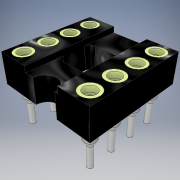
# Autodesk Inventor part: DIL8-Socket
Saved by Autodesk Inventor 2018 (Build 220112000, 112)
## iProperties
Created: 2020-04-18
Part Number: DIL8-Socket
Material: Všeobecné
Document SubType Name: Modeling
Designer: Jozko Mrkvicka
Density: 1 g/cm^3
Appearance: Výchozí
Author: Jozko Mrkvicka
Autodesk Inventor part; units mm, degrees
ref_plane "YZ Plane" through (0, 0, 0) normal (1, 0, 0) x (0, 1, 0)
ref_plane "XZ Plane" through (0, 0, 0) normal (0, 1, 0) x (-1, 0, 0)
ref_plane "XY Plane" through (0, 0, 0) normal (0, 0, 1) x (1, 0, 0)
sketch "Náčrt1" plane through (0, 0, 0) normal (0, 1, 0) x (-1, 0, 0)
  line L0 (10.16, 0) -> (10.16, -10.16)
  line L1 (10.16, -10.16) -> (0, -10.16)
  line L2 (0, -10.16) -> (0, 0)
  line L3 (0, 0) -> (3.175, 0)
  line L4 (3.175, -10.16) -> (0, -10.16)
  line L5 (0, -10.16) -> (0, 0)
  line L6 (10.16, 0) -> (6.985, 0)
  line L7 (6.985, -10.16) -> (10.16, -10.16)
  line L8 (10.16, -10.16) -> (10.16, 0)
  line L9 (3.81, -3.175) -> (6.35, -3.175)
  line L10 (6.985, -10.16) -> (3.175, -10.16)
  line L11 (3.81, -6.985) -> (6.35, -6.985)
  line L12 (6.985, -3.81) -> (6.985, -6.35)
  line L13 (3.175, -3.81) -> (3.175, -6.35)
  arc A0 (3.4925, 0) -> (6.0325, 0) centre (4.7625, 0) ccw
  line L14 (0, 0) -> (3.4925, 0)
  line L15 (6.0325, 0) -> (10.16, 0)
  line L16 (6.985, 0) -> (6.0325, 0)
  line L17 (3.4925, 0) -> (3.175, 0)
  arc A1 (6.985, -3.81) -> (6.35, -3.175) centre (6.35, -3.81) ccw
  arc A2 (3.81, -3.175) -> (3.175, -3.81) centre (3.81, -3.81) ccw
  arc A3 (3.175, -6.35) -> (3.81, -6.985) centre (3.81, -6.35) ccw
  arc A4 (6.35, -6.985) -> (6.985, -6.35) centre (6.35, -6.35) ccw
  dimension "d0" = 10.16
  dimension "d1" = 10.16
  dimension "d6" = 2.54
  dimension "d7" = 0.635
  dimension "d111" = 3.175
  dimension "d112" = 3.175
  constraints: 36 end point, 10 point on circle, 9 parallel, 8 horizontal, 8 tangent, 5 centre point, 4 perpendicular, 3 equal radius, 2 point on line
  measures "d0" distance of L0.end L1.end
  measures "d1" distance of L0.start L0.end
  measures "d6" diameter of A0
  measures "d7" radius of A1
  measures "d111" distance between parallel lines of L1 L11
  measures "d112" distance between parallel lines of L3 L9
extrude "Vysunutí15" add sketch "Náčrt1" along normal blind 3.175
sketch "Náčrt14" plane through (0, 3.175, 0) normal (0, 1, 0) x (1, 0, 0)
  line L0 (-6.985, 11.6552) -> (-3.175, 11.6552)
  line L1 (-3.175, 11.6552) -> (-3.175, -1.5875)
  line L2 (-3.175, -1.5875) -> (-6.985, -1.5875)
  line L3 (-6.985, -1.5875) -> (-6.985, 11.6552)
  point P0 (0, 0)
  constraints: 8 end point, 2 parallel, 1 horizontal, 1 perpendicular
extrude "Vysunutí16" cut sketch "Náčrt14" against normal blind 0.635
sketch "Náčrt15" plane through (0, 3.175, 0) normal (0, 1, 0) x (1, 0, 0)
  circle A0 centre (-8.89, 8.89) radius 0.635
  circle A1 centre (-8.89, 6.35) radius 0.635
  circle A2 centre (-8.89, 3.81) radius 0.635
  circle A3 centre (-8.89, 1.27) radius 0.635
  circle A4 centre (-1.27, 8.89) radius 0.635
  circle A5 centre (-1.27, 6.35) radius 0.635
  circle A6 centre (-1.27, 3.81) radius 0.635
  circle A7 centre (-1.27, 1.27) radius 0.635
  point P0 (0, 0)
  point P1 (0, 0)
  point P2 (-1.27, 8.89)
  point P3 (-1.27, 6.35)
  point P4 (-1.27, 3.81)
  point P5 (-1.27, 1.27)
  point P6 (-8.89, 1.27)
  point P7 (-8.89, 3.81)
  point P8 (-8.89, 6.35)
  point P9 (-8.89, 8.89)
  point P10 (-1.27, 1.27)
  constraints: 8 centre point
extrude "Vysunutí17" cut sketch "Náčrt15" against normal blind 0.635
sketch "Náčrt16" plane through (-8.89, 2.54, -1.27) normal (0, 1, 0) x (1, 0, 0)
  circle A0 centre (0, 7.62) radius 0.3175
  circle A1 centre (0, 7.62) radius 0.3175
  circle A2 centre (7.62, 5.08) radius 0.3175
  circle A3 centre (7.62, 5.08) radius 0.3175
  circle A4 centre (7.62, 2.54) radius 0.3175
  circle A5 centre (7.62, 0) radius 0.3175
  circle A6 centre (7.62, 0) radius 0.3175
  circle A7 centre (0, 5.08) radius 0.3175
  circle A8 centre (0, 2.54) radius 0.3175
  circle A9 centre (0, 0) radius 0.3175
  circle A10 centre (0, 0) radius 0.3175
  circle A11 centre (7.62, 7.62) radius 0.3175
  point P0 (8.89, -1.27)
  point P1 (8.89, -1.27)
  constraints: 12 centre point, 8 coincident
extrude "Vysunutí18" cut sketch "Náčrt16" against normal blind 1.27
sketch "Náčrt17" plane through (0, 3.175, 0) normal (0, 1, 0) x (1, 0, 0)
  circle A0 centre (-8.89, 1.27) radius 0.9525
  circle A1 centre (-8.89, 8.89) radius 0.9525
  circle A2 centre (-8.89, 3.81) radius 0.9525
  circle A3 centre (-8.89, 6.35) radius 0.9525
  circle A4 centre (-1.27, 8.89) radius 0.9525
  circle A5 centre (-1.27, 3.81) radius 0.9525
  circle A6 centre (-1.27, 1.27) radius 0.9525
  circle A7 centre (-1.27, 6.35) radius 0.9525
  point P0 (0, 0)
  constraints: 8 centre point
extrude "Vysunutí19" cut sketch "Náčrt17" against normal blind 0.0254
sketch "Náčrt18" plane through (0, 0, 0) normal (0, -1, 0) x (1, 0, 0)
  circle A0 centre (-1.27, -8.89) radius 0.635 projected
  circle A1 centre (-1.27, -6.35) radius 0.635 projected
  circle A2 centre (-1.27, -3.81) radius 0.635 projected
  circle A3 centre (-1.27, -1.27) radius 0.635 projected
  circle A4 centre (-8.89, -8.89) radius 0.635 projected
  circle A5 centre (-8.89, -6.35) radius 0.635 projected
  circle A6 centre (-8.89, -3.81) radius 0.635 projected
  circle A7 centre (-8.89, -1.27) radius 0.635 projected
  point P0 (0, 0)
extrude "Vysunutí20" add sketch "Náčrt18" along normal blind 1.905
chamfer "Zkosení45" distance 0.3175 distance2 0.635 1 edges at (-9.525, -1.905, -8.89) measured on face at (-8.6783, -1.905, -9.0867)
chamfer "Zkosení46" distance 0.3175 distance2 0.635 1 edges at (-9.525, -1.905, -6.35) measured on face at (-8.6964, -1.905, -6.499)
chamfer "Zkosení47" distance 0.3175 distance2 0.635 1 edges at (-9.525, -1.905, -3.81) measured on face at (-8.6964, -1.905, -3.959)
chamfer "Zkosení48" distance 0.3175 distance2 0.635 1 edges at (-9.525, -1.905, -1.27) measured on face at (-8.6964, -1.905, -1.419)
chamfer "Zkosení49" distance 0.3175 distance2 0.635 1 edges at (-1.905, -1.905, -8.89) measured on face at (-1.4636, -1.905, -8.9377)
chamfer "Zkosení50" distance 0.3175 distance2 0.635 1 edges at (-1.905, -1.905, -6.35) measured on face at (-1.0645, -1.905, -6.4007)
chamfer "Zkosení51" distance 0.3175 distance2 0.635 1 edges at (-1.905, -1.905, -3.81) measured on face at (-1.0282, -1.905, -4.0079)
chamfer "Zkosení52" distance 0.3175 distance2 0.635 1 edges at (-1.905, -1.905, -1.27) measured on face at (-1.0935, -1.905, -1.2787)
sketch "Náčrt19" plane through (-8.89, -1.905, -8.89) normal (0, -1, 0) x (1, 0, 0)
  circle A0 centre (0, 7.62) radius 0.3175 projected
  circle A1 centre (0, 5.08) radius 0.3175 projected
  circle A2 centre (0, 2.54) radius 0.3175 projected
  circle A3 centre (0, 0) radius 0.3175 projected
  circle A4 centre (7.62, 7.62) radius 0.3175 projected
  circle A5 centre (7.62, 5.08) radius 0.3175 projected
  circle A6 centre (7.62, 2.54) radius 0.3175 projected
  circle A7 centre (7.62, 0) radius 0.3175 projected
  point P0 (8.89, 8.89)
extrude "Vysunutí21" add sketch "Náčrt19" along normal blind 2.54
fillet "Zaoblení3" radius 0.127 8 edges at (-1.5875, -4.445, -1.27) (-1.5875, -4.445, -3.81) (-1.5875, -4.445, -6.35) (-1.5875, -4.445, -8.89) (-9.2075, -4.445, -1.27) (-9.2075, -4.445, -3.81) (-9.2075, -4.445, -6.35) (-9.2075, -4.445, -8.89)
